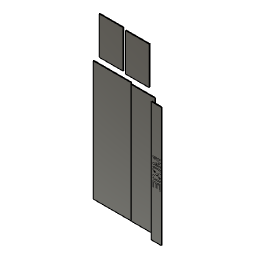
Mixie (Autodesk Fusion 360 design; units mm, degrees)
Autodesk Fusion 360 part; units mm, degrees
sketch "Sketch1" plane through (0, 0, 0) normal (0, 0, 1) x (1, 0, 0)
  line L0 (-110, 175) -> (110, 175)
  line L1 (110, 175) -> (110, -175)
  line L2 (110, -175) -> (-110, -175)
  line L3 (-110, -175) -> (-110, 175)
  line L4 (-110, 175) -> (110, -175) construction
  line L5 (110, 175) -> (-110, -175) construction
  dimension "d1" = 220
  dimension "d2" = 350
  constraint horizontal L0
  constraint perpendicular L0 L1
  constraint parallel L0 L2
  constraint parallel L1 L3
  constraint coincident L4 origin
  constraint coincident L5 origin
  measures "d1" distance of L1.end L2.end
  measures "d2" distance of L0.end L1.end
extrude "Extrude1" add sketch "Sketch1" along normal blind 6 makes body 1
extrude "Extrude2" add sketch "Sketch1" along normal blind 6 separate body makes body 2
sketch "Sketch2" plane through (0, 0, 6) normal (0, 0, 1) x (-1, 0, 0)
  line L0 (110, 175) -> (-110, 175)
  line L1 (-110, 175) -> (-110, -175)
  line L2 (-110, -175) -> (110, -175)
  line L3 (110, -175) -> (110, 175)
  line L4 (-110, 0) -> (-110, -87.5)
  line L5 (-110, -87.5) -> (110, -87.5)
  line L6 (110, -87.5) -> (110, -81.5)
  line L7 (-110, -87.5) -> (-110, -81.5)
  line L8 (110, -81.5) -> (-110, -81.5)
  dimension "d8" = 87.5
  dimension "d9" = 6
  dimension "d10" = 6
  constraint midpoint L1 L4.start
  constraint perpendicular L2 L4
  constraint coincident L3 L5.end
  constraint perpendicular L3 L5
  constraint perpendicular L5 L6
  constraint perpendicular L5 L7
  measures "d8" distance of L4.start L4.end
  measures "d9" distance of L5.end L6.end
  measures "d10" distance of L4.end L7.end
extrude "Extrude3" add sketch "Sketch2" along normal blind 1100 separate body contours L1 L3 L4 L5 L6 L7 L8 makes body 3
extrude "Extrude4" add sketch "Sketch1" along normal blind 6 from surface at 1106 separate body makes body 4
sketch "Sketch4" plane through (-110, 0, 0) normal (-1, 0, 0) x (0, -1, 0)
  line L0 (175, 0) -> (175, 1112)
  line L1 (175, 1112) -> (-175, 1112)
  line L2 (-175, 1112) -> (-175, 0)
  line L3 (-175, 0) -> (175, 0)
  dimension "d34" = 1112
  constraint perpendicular L0 L1
  constraint parallel L0 L2
  constraint parallel L1 L3
  constraint vertical L0
  measures "d34" distance of L0.start L0.end
extrude "Extrude6" add sketch "Sketch4" along normal blind 6 separate body makes body 5
sketch "Sketch5" plane through (0, 87.5, 0) normal (0, 1, 0) x (-1, 0, 0)
  line L0 (110, 6) -> (110, 1106)
  line L1 (110, 1106) -> (-110, 1106)
  line L2 (-110, 1106) -> (-110, 6)
  line L3 (0, 976.5) -> (0, 869.5)
  line L4 (0, 854.5) -> (0, 747.5)
  circle A0 centre (0, 984) radius 7.5
  circle A1 centre (0, 862) radius 7.5
  circle A2 centre (0, 740) radius 7.5
  line L5 (0, 732.5) -> (0, 625.5)
  line L6 (0, 610.5) -> (0, 503.5)
  circle A3 centre (0, 618) radius 7.5
  line L7 (-110, 6) -> (110, 6)
  line L8 (0, 488.5) -> (0, 381.5)
  line L9 (0, 366.5) -> (0, 259.5)
  line L10 (0, 244.5) -> (0, 137.5)
  line L11 (0, 122.5) -> (0, 8)
  line L12 (0, 1106) -> (0, 984)
  circle A4 centre (0, 496) radius 7.5
  circle A5 centre (0, 374) radius 7.5
  circle A6 centre (0, 252) radius 7.5
  circle A7 centre (0, 130) radius 7.5
  dimension "d22" = 122
  dimension "d23" = 122
  dimension "d25" = 15
  dimension "d26" = 15
  dimension "d27" = 15
  dimension "d28" = 122
  dimension "d29" = 122
  dimension "d30" = 15
  dimension "d154" = 122
  dimension "d155" = 122
  dimension "d156" = 122
  dimension "d157" = 122
  dimension "d160" = 122
  dimension "d161" = 15
  dimension "d162" = 15
  dimension "d163" = 15
  dimension "d164" = 15
  constraint parallel L3 L4
  constraint parallel L4 L5
  constraint parallel L5 L6
  constraint coincident A0 L3.start
  constraint coincident A1 L3.end
  constraint coincident A1 L4.start
  constraint coincident A2 L4.end
  constraint coincident A2 L5.start
  constraint coincident A3 L5.end
  constraint coincident A3 L6.start
  constraint parallel L6 L8
  constraint parallel L8 L9
  constraint parallel L9 L10
  constraint parallel L10 L11
  constraint midpoint L1 L12.start
  constraint coincident A0.centre L12.end
  constraint perpendicular L1 L12
  constraint coincident A5 L8.end
  constraint coincident A5 L9.start
  constraint coincident A6 L10.start
  constraint coincident A6 L9.end
  constraint coincident A7 L11.start
  constraint coincident A7 L10.end
  constraint coincident A4 L8.start
  constraint coincident A4 L6.end
  measures "d22" distance of A0.centre A1.centre
  measures "d23" distance of A1.centre A2.centre
  measures "d25" diameter of A0
  measures "d26" diameter of A1
  measures "d27" diameter of A2
  measures "d28" distance of A2.centre A3.centre
  measures "d29" distance of A3.centre A4.centre
  measures "d30" diameter of A3
  measures "d154" distance of A4.centre A5.centre
  measures "d155" distance of A5.centre A6.centre
  measures "d156" distance of A6.centre A7.centre
  measures "d157" distance of L11.end A7.centre
  measures "d160" distance of L12.start A0.centre
  measures "d161" diameter of A4
  measures "d162" diameter of A5
  measures "d163" diameter of A6
  measures "d164" diameter of A7
sketch "Sketch6" plane through (110, 0, 0) normal (1, 0, 0) x (0, 1, 0)
  line L0 (81.5, 6) -> (87.5, 6)
  line L1 (87.5, 6) -> (87.5, 1106)
  line L2 (87.5, 1106) -> (81.5, 1106)
  line L3 (81.5, 1106) -> (81.5, 6)
  line L4 (81.5, 1106) -> (81.5, 1112)
  line L5 (81.5, 1112) -> (175, 1112)
  line L6 (175, 1112) -> (175, 0)
  line L7 (175, 0) -> (81.5, 0)
  line L8 (81.5, 0) -> (81.5, 1112)
  constraint coincident L2.end L3.start
  constraint perpendicular L2 L4
  constraint perpendicular L5 L6
  constraint parallel L5 L7
  constraint parallel L6 L8
  constraint perpendicular L4 L5
extrude "Extrude8" add sketch "Sketch6" along normal blind 6 separate body makes body 6
sketch "Sketch7" plane through (116, 0, 0) normal (1, 0, 0) x (0, 1, 0)
  line L0 (81.5, 0) -> (175, 0)
  line L1 (175, 0) -> (175, 1112)
  line L2 (175, 1112) -> (81.5, 1112)
  line L3 (81.5, 1112) -> (81.5, 0)
  line L4 (81.5, 1112) -> (81.5, 0) construction
  line L5 (81.5, 0) -> (175, 0) construction
  line L6 (175, 0) -> (175, 1112) construction
  line L7 (175, 1112) -> (81.5, 1112) construction
  dimension "d151" = 70
  text T0 "MIXIE" font "Arial" height 70 align centre middle in box 1112 x 93.5 at (81.5, 1112) x (0, -1) y (1, 0) spacing 1
  constraint coincident L0.start
  constraint coincident L1.end
extrude "Extrude15" cut sketch "Sketch7" against normal blind 1 text T0 bodies 6
copy_body "CopyPasteBodies1" bodies 1 2 3 4 5 6 makes body 7 makes body 8 makes body 9 makes body 10 makes body 11 makes body 12
move_body "Move1" bodies 7 8 9 10 11 12 to x (1, 0, 0) y (0, 1, 0) z (0, 0, 1) at (1000, 0, 0)
move_body "Move2" bodies 11 to x (0, 1, 0) y (-1, 0, 0) z (0, 0, 1) at (715, -1065, 0)
move_body "Move3" bodies 10 to x (1, 0, 0) y (0, 0, 1) z (0, -1, 0) at (0, 937, 1287)
move_body "Move4" bodies 10 to x (1, 0, 0) y (0, 1, 0) z (0, 0, 1) at (-300, 0, 50)
move_body "Move5" bodies 9 to x (1, 0, 0) y (0, 1, 0) z (0, 0, 1) at (0, -270, 0)
move_body "Move6" bodies 8 to x (1, 0, 0) y (0, 0, -1) z (0, 1, 0) at (0, -181, -169)
delete_body "RemoveBody1" bodies 7
move_body "Move7" bodies 9 to x (1, 0, 0) y (0, 1, 0) z (0, 0, 1) at (10, 0, 0)
move_body "Move8" bodies 8 to x (1, 0, 0) y (0, 1, 0) z (0, 0, 1) at (-50, 0, 1500)
move_body "Move9" bodies 12 to x (0, 1, 0) y (-1, 0, 0) z (0, 0, 1) at (1252.7016, -1349.2984, 0)
move_body "Move10" bodies 12 to x (1, 0, 0) y (0, 1, 0) z (0, 0, 1) at (10, 0, 0)
move_body "Move11" bodies 12 to x (1, 0, 0) y (0, 1, 0) z (0, 0, 1) at (50, 0, 0)
hidden bodies 1 2 3 4 5 6
equation "þykkt = 6 mm"
equation "d4 = þykkt"
equation "d6 = þykkt"
equation "d8 = ( 175 / 2 ) * 1 mm"
equation "d9 = þykkt"
equation "d10 = þykkt"
equation "d18 = þykkt"
equation "gat = 15 mm"
equation "d25 = gat"
equation "d26 = gat"
equation "d27 = gat"
equation "d30 = gat"
equation "lengd = 400 mm"
equation "d35 = þykkt"
equation "d161 = gat"
equation "d162 = gat"
equation "d163 = gat"
equation "d164 = gat"
